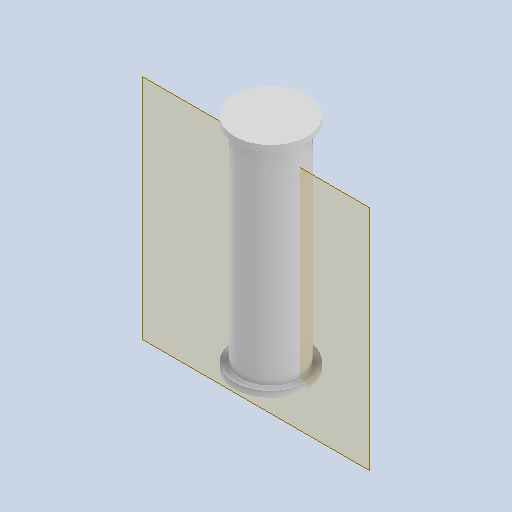
# Autodesk Inventor part: nitR1
Saved by Autodesk Inventor 2025 (Build 290162000, 162)
## iProperties
Created: 2025-02-05
Part Number: nitR1
Material: Generic
Document SubType Name: Modeling
Designer: piotr
Density: 1 g/cm^3
Appearance: Default
Author: piotr
Autodesk Inventor part; units mm, degrees
ref_plane "YZ Plane" through (0, 0, 0) normal (1, 0, 0) x (0, 1, 0)
ref_plane "XZ Plane" through (0, 0, 0) normal (0, 1, 0) x (-1, 0, 0)
ref_plane "XY Plane" through (0, 0, 0) normal (0, 0, 1) x (1, 0, 0)
ref_plane "Work Plane1" through (5, 35, -37.5) normal (0, 0, 1) x (1, 0, 0)
sketch "Sketch1" plane through (5, 35, -37.5) normal (0, 0, 1) x (1, 0, 0)
  line L0 (-10, 11.7937) -> (10, 11.7937) projected
  line L1 (10, 11.7937) -> (10, -58.2063)
  line L2 (10, -58.2063) -> (12.25, -58.2063)
  line L3 (12.25, -58.2063) -> (12.25, -60.2063)
  line L4 (12.25, -60.2063) -> (-12.25, -60.2063)
  line L5 (-12.25, -60.2063) -> (-12.25, -58.2063)
  line L6 (-12.25, -58.2063) -> (-10, -58.2063)
  line L7 (-10, -58.2063) -> (-10, 11.7937)
  line L8 (-10, 11.7937) -> (-12.25, 11.7937)
  line L9 (-12.25, 11.7937) -> (-12.25, 13.7937)
  line L10 (-12.25, 13.7937) -> (12.25, 13.7937)
  line L11 (12.25, 13.7937) -> (12.25, 11.7937)
  line L12 (12.25, 11.7937) -> (10, 11.7937)
  line L13 (0, 29.0063) -> (0, -66.419)
  point P0 (-5, -35)
  point P1 (0, 11.7937)
  point P2 (0, 13.7937)
  point P3 (0, -60.2063)
  dimension "d0" = 2.25
  dimension "d1" = 70
  dimension "d2" = 2
  dimension "d3" = 24.5
  dimension "d4" = 2
  dimension "d5" = 2.25
  dimension "d6" = 70
  dimension "d7" = 2.25
  dimension "d8" = 2
  dimension "d9" = 24.5
  dimension "d10" = 2
  constraints: 26 end point, 5 perpendicular, 3 point on line, 3 vertical, 1 horizontal, 1 midpoint
  measures "d0" distance of L1.end L2.end
  measures "d1" distance of L0.end L1.end
  measures "d2" distance of L2.end L3.end
  measures "d3" distance of L3.end L4.end
  measures "d4" distance of L4.end L5.end
  measures "d5" distance of L5.end L6.end
  measures "d6" distance of L6.end L0.start
  measures "d7" distance of L0.start L8.end
  measures "d8" distance of L8.end L9.end
  measures "d9" distance of L9.end L10.end
  measures "d10" distance of L10.end L11.end
revolve "Revolution1" add sketch "Sketch1" angle 360 about axis through (5, 64.0063, -37.5) along (0, -1, 0) contours L13 L10 L11 L12 L0 | L0 L1 L2 L3 L4 L13
body "Solid1"
